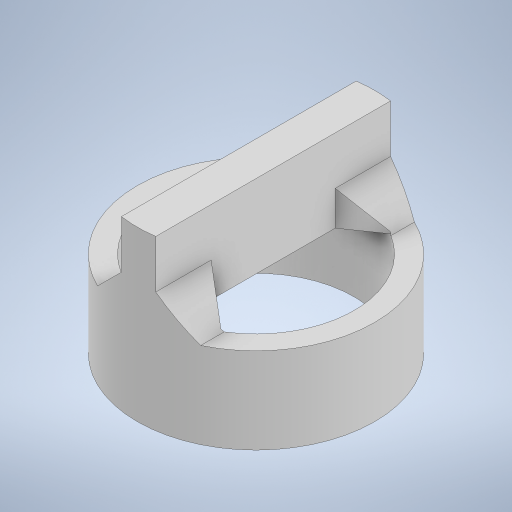
# Autodesk Inventor part: terminalcap_4.1mm_addon
Saved by Autodesk Inventor 2024 (Build 280153000, 153)
## iProperties
Created: 2024-04-25
Part Number: terminalcap_4.1mm_addon
Material: 일반
Document SubType Name: Modeling
Designer: Gihyeok Na
Density: 1 g/cm^3
Appearance: 기본값
Author: Gihyeok Na
Autodesk Inventor part; units mm, degrees
ref_plane "YZ Plane" through (0, 0, 0) normal (1, 0, 0) x (0, 1, 0)
ref_plane "XZ Plane" through (0, 0, 0) normal (0, 1, 0) x (-1, 0, 0)
ref_plane "XY Plane" through (0, 0, 0) normal (0, 0, 1) x (1, 0, 0)
sketch "스케치1" plane through (0, 0, 0) normal (0, 1, 0) x (-1, 0, 0)
  circle A0 centre (0, 0) radius 2.85
  circle A1 centre (0, 0) radius 3.45
  dimension "d0" = 5.7
  dimension "d1" = 6.9
  constraints: 2 centre point, 2 coincident
  measures "d0" diameter of A0
  measures "d1" diameter of A1
extrude "돌출1" add sketch "스케치1" along normal blind 2.5
sketch "스케치2" plane through (0, 2.5, 0) normal (0, 1, 0) x (1, 0, 0)
  circle A0 centre (0, 0) radius 3.45 projected
  circle A1 centre (0, 0) radius 3.45 projected
  line L0 (0.5, 3.4136) -> (-0.5, 3.4136)
  line L1 (-0.5, 3.4136) -> (-0.5, -3.4136)
  line L2 (-0.5, -3.4136) -> (0.5, -3.4136)
  line L3 (0.5, -3.4136) -> (0.5, 3.4136)
  line L4 (0.5, 3.4136) -> (-0.5, -3.4136) construction
  line L5 (-0.5, 3.4136) -> (0.5, -3.4136) construction
  point P0 (-0.5, -3.4136)
  point P1 (0.5, -3.4136)
  point P2 (0.5, 3.4136)
  point P3 (-0.5, 3.4136)
  dimension "d4" = 1
  constraints: 12 end point, 2 midpoint, 2 parallel, 1 horizontal, 1 perpendicular, 1 point on circle
  measures "d4" distance of L2.end L1.end
extrude "돌출2" add sketch "스케치2" along normal blind 2.4 contours L0 A0 | L3 L2 L1 L0 | A0 L2
chamfer "모따기1" distance 1 angle 45 4 edges at (0.5, 2.5, 3.1097) (0.5, 2.5, -3.1097) (-0.5, 2.5, -3.1097) (-0.5, 2.5, 3.1097)
chamfer "모따기2" distance 1 angle 45 4 edges at (-0.5, 3, -2.8058) (-0.5, 3, 2.8058) (0.5, 3, 2.8058) (0.5, 3, -2.8058)
